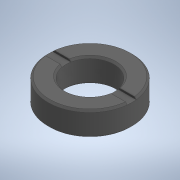
# Autodesk Inventor part: GSB-081404
Saved by Autodesk Inventor 2020 (Build 240168000, 168)
## iProperties
Created: 2021-08-03
Part Number: GSB-081404
Material: 一般
Document SubType Name: Modeling
Designer: naoki
Density: 1 g/cm^3
Appearance: 既定
Author: naoki
Autodesk Inventor part; units mm, degrees
ref_plane "YZ Plane" through (0, 0, 0) normal (1, 0, 0) x (0, 1, 0)
ref_plane "XZ Plane" through (0, 0, 0) normal (0, 1, 0) x (-1, 0, 0)
ref_plane "XY Plane" through (0, 0, 0) normal (0, 0, 1) x (1, 0, 0)
sketch "スケッチ1" plane through (0, 0, 0) normal (0, 1, 0) x (-1, 0, 0)
  circle A0 centre (0, 0) radius 7
  circle A1 centre (0, 0) radius 4
  dimension "d0" = 14
  dimension "d1" = 8
  constraints: 2 centre point, 2 coincident
  measures "d0" diameter of A0
  measures "d1" diameter of A1
extrude "押し出し1" add sketch "スケッチ1" along normal blind 4
sketch "スケッチ2" plane through (0, 4, 0) normal (0, 1, 0) x (1, 0, 0)
  circle A0 centre (0, 0) radius 7 projected
  line L0 (-7, 0) -> (7, 0)
  line L1 (-7, 0.75) -> (7, 0.75)
  line L2 (-7, 0.75) -> (-7, 0)
  line L3 (7, 0.75) -> (7, 0)
  line L4 (-7, -0.75) -> (7, -0.75)
  line L5 (-7, -0.75) -> (-7, 0)
  line L6 (7, -0.75) -> (7, 0)
  point P0 (6.9597, 0.75)
  point P1 (-6.9597, 0.75)
  point P2 (-6.9597, -0.75)
  point P3 (6.9597, -0.75)
  dimension "d4" = 0.75
  constraints: 14 end point, 2 parallel, 2 point on circle, 2 symmetric about line, 2 tangent, 1 horizontal, 1 vertical
  measures "d4" distance between parallel lines of L0 L1
extrude "押し出し2" cut sketch "スケッチ2" against normal blind 0.3 contours L0 A0 L1 | A0 L4 L0
chamfer "面取り1" distance 0.3 angle 45 6 edges at (0, 4, 4) (0, 4, -4) (0, 4, -7) (0, 4, 7) (7, 0, 0) (4, 0, 0)
